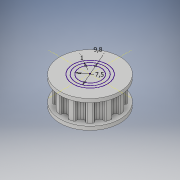
# Autodesk Inventor part: BeltPulleyT5_12Z
Saved by Autodesk Inventor 2018.3 (Build 223284000, 284)
## iProperties
Created: 2018-07-24
Part Number: BeltPulleyT5_12Z
Material: Generisch
Document SubType Name: Modeling
Designer: JochenAlt
Density: 1 g/cm^3
Appearance: Vorgabe
Author: JochenAlt
Autodesk Inventor part; units mm, degrees
ref_plane "YZ Plane" through (0, 0, 0) normal (1, 0, 0) x (0, 1, 0)
ref_plane "XZ Plane" through (0, 0, 0) normal (0, 1, 0) x (-1, 0, 0)
ref_plane "XY Plane" through (0, 0, 0) normal (0, 0, 1) x (1, 0, 0)
sketch "Skizze1" plane through (0, 0, 0) normal (0, 0, 1) x (1, 0, 0)
  circle A0 centre (0, 0) radius 3.75
  dimension "d0" = 7.5
  constraints: 1 centre point, 1 coincident
  measures "d0" diameter of A0
sketch "Skizze9" plane through (0, 0, 0) normal (1, 0, 0) x (0, 1, 0)
  line L0 (0, 0) -> (0, -14)
  line L1 (0, 0) -> (-10.325, 0)
  line L2 (-10.325, 0) -> (-10.325, -1.25)
  line L3 (-10.325, -1.25) -> (-9.125, -1.25)
  line L4 (-9.125, -1.25) -> (-9.125, -8.25)
  line L5 (-9.125, -8.25) -> (-10.325, -8.25)
  line L6 (-10.325, -8.25) -> (-10.325, -9.5)
  line L7 (-10.325, -9.5) -> (0, -9.5)
  line L8 (0, -9.5) -> (0, 0)
  dimension "d56" = 1.25
  dimension "d57" = 10.325
  dimension "d58" = 1.2
  dimension "d62" = 0
  dimension "d75" = 7
  constraints: 18 end point, 4 perpendicular, 2 collinear, 2 point on line, 2 vertical, 1 coincident, 1 horizontal, 1 parallel
  measures "d56" distance of L1.end L2.end
  measures "d57" distance of L0.start L1.end
  measures "d58" distance of L2.end L3.end
  measures "d62" distance between parallel lines of L0 L8
  measures "d75" distance of L3.end L4.end
revolve "Umdrehung5" add sketch "Skizze9" angle 360 about axis through (0, 0, 0) along (0, 0, -1)
sketch "Skizze10" plane through (0, 0, -1.25) normal (0, 0, -1) x (-1, 0, 0)
  circle A0 centre (0, 0) radius 36.5
  arc A1 (-8.9649, 1.7016) -> (-8.7088, 1.2512) centre (-8.572, 1.627) ccw
  line L0 (-8.7088, 1.2512) -> (-8.1066, 1.032)
  arc A2 (-7.7128, 0.4344) -> (-8.1066, 1.032) centre (-8.3118, 0.4682) ccw
  arc A3 (-7.7128, 0.4344) -> (-7.7128, -0.4344) centre (0, 0) ccw
  arc A4 (-8.1066, -1.032) -> (-7.7128, -0.4344) centre (-8.3118, -0.4682) ccw
  line L1 (-8.1066, -1.032) -> (-8.7088, -1.2512)
  arc A5 (-8.7088, -1.2512) -> (-8.9649, -1.7016) centre (-8.572, -1.627) ccw
  arc A6 (-8.9649, -1.7016) -> (-8.8141, -2.3617) centre (0, 0) ccw
  arc A7 (-8.8141, -2.3617) -> (-8.6147, -3.0088) centre (0, 0) ccw
  arc A8 (-8.6147, -3.0088) -> (-8.1676, -3.2708) centre (-8.237, -2.8769) ccw
  line L2 (-8.1676, -3.2708) -> (-7.5365, -3.1596)
  arc A9 (-6.8967, -3.4802) -> (-7.5365, -3.1596) centre (-7.4323, -3.7505) ccw
  arc A10 (-6.8967, -3.4802) -> (-6.4622, -4.2326) centre (0, 0) ccw
  arc A11 (-6.5045, -4.947) -> (-6.4622, -4.2326) centre (-6.9642, -4.5614) ccw
  line L3 (-6.5045, -4.947) -> (-6.9164, -5.4379)
  arc A12 (-6.9164, -5.4379) -> (-6.9131, -5.9561) centre (-6.61, -5.695) ccw
  arc A13 (-6.9131, -5.9561) -> (-6.4523, -6.4523) centre (0, 0) ccw
  arc A14 (-6.4523, -6.4523) -> (-5.9561, -6.9131) centre (0, 0) ccw
  arc A15 (-5.9561, -6.9131) -> (-5.4379, -6.9164) centre (-5.695, -6.61) ccw
  line L4 (-5.4379, -6.9164) -> (-4.947, -6.5045)
  arc A16 (-4.2326, -6.4622) -> (-4.947, -6.5045) centre (-4.5614, -6.9642) ccw
  arc A17 (-4.2326, -6.4622) -> (-3.4802, -6.8967) centre (0, 0) ccw
  arc A18 (-3.1596, -7.5365) -> (-3.4802, -6.8967) centre (-3.7505, -7.4323) ccw
  line L5 (-3.1596, -7.5365) -> (-3.2708, -8.1676)
  arc A19 (-3.2708, -8.1676) -> (-3.0088, -8.6147) centre (-2.8769, -8.237) ccw
  arc A20 (-3.0088, -8.6147) -> (-2.3617, -8.8141) centre (0, 0) ccw
  arc A21 (-2.3617, -8.8141) -> (-1.7016, -8.9649) centre (0, 0) ccw
  arc A22 (-1.7016, -8.9649) -> (-1.2512, -8.7088) centre (-1.627, -8.572) ccw
  line L6 (-1.2512, -8.7088) -> (-1.032, -8.1066)
  arc A23 (-0.4344, -7.7128) -> (-1.032, -8.1066) centre (-0.4682, -8.3118) ccw
  arc A24 (-0.4344, -7.7128) -> (0.4344, -7.7128) centre (0, 0) ccw
  arc A25 (1.032, -8.1066) -> (0.4344, -7.7128) centre (0.4682, -8.3118) ccw
  line L7 (1.032, -8.1066) -> (1.2512, -8.7088)
  arc A26 (1.2512, -8.7088) -> (1.7016, -8.9649) centre (1.627, -8.572) ccw
  arc A27 (1.7016, -8.9649) -> (2.3617, -8.8141) centre (0, 0) ccw
  arc A28 (2.3617, -8.8141) -> (3.0088, -8.6147) centre (0, 0) ccw
  arc A29 (3.0088, -8.6147) -> (3.2708, -8.1676) centre (2.8769, -8.237) ccw
  line L8 (3.2708, -8.1676) -> (3.1596, -7.5365)
  arc A30 (3.4802, -6.8967) -> (3.1596, -7.5365) centre (3.7505, -7.4323) ccw
  arc A31 (3.4802, -6.8967) -> (4.2326, -6.4622) centre (0, 0) ccw
  arc A32 (4.947, -6.5045) -> (4.2326, -6.4622) centre (4.5614, -6.9642) ccw
  line L9 (4.947, -6.5045) -> (5.4379, -6.9164)
  arc A33 (5.4379, -6.9164) -> (5.9561, -6.9131) centre (5.695, -6.61) ccw
  arc A34 (5.9561, -6.9131) -> (6.4523, -6.4523) centre (0, 0) ccw
  arc A35 (6.4523, -6.4523) -> (6.9131, -5.9561) centre (0, 0) ccw
  arc A36 (6.9131, -5.9561) -> (6.9164, -5.4379) centre (6.61, -5.695) ccw
  line L10 (6.9164, -5.4379) -> (6.5045, -4.947)
  arc A37 (6.4622, -4.2326) -> (6.5045, -4.947) centre (6.9642, -4.5614) ccw
  arc A38 (6.4622, -4.2326) -> (6.8967, -3.4802) centre (0, 0) ccw
  arc A39 (7.5365, -3.1596) -> (6.8967, -3.4802) centre (7.4323, -3.7505) ccw
  line L11 (7.5365, -3.1596) -> (8.1676, -3.2708)
  arc A40 (8.1676, -3.2708) -> (8.6147, -3.0088) centre (8.237, -2.8769) ccw
  arc A41 (8.6147, -3.0088) -> (8.8141, -2.3617) centre (0, 0) ccw
  arc A42 (8.8141, -2.3617) -> (8.9649, -1.7016) centre (0, 0) ccw
  arc A43 (8.9649, -1.7016) -> (8.7088, -1.2512) centre (8.572, -1.627) ccw
  line L12 (8.7088, -1.2512) -> (8.1066, -1.032)
  arc A44 (7.7128, -0.4344) -> (8.1066, -1.032) centre (8.3118, -0.4682) ccw
  arc A45 (7.7128, -0.4344) -> (7.7128, 0.4344) centre (0, 0) ccw
  arc A46 (8.1066, 1.032) -> (7.7128, 0.4344) centre (8.3118, 0.4682) ccw
  line L13 (8.1066, 1.032) -> (8.7088, 1.2512)
  arc A47 (8.7088, 1.2512) -> (8.9649, 1.7016) centre (8.572, 1.627) ccw
  arc A48 (8.9649, 1.7016) -> (8.8141, 2.3617) centre (0, 0) ccw
  arc A49 (8.8141, 2.3617) -> (8.6147, 3.0088) centre (0, 0) ccw
  arc A50 (8.6147, 3.0088) -> (8.1676, 3.2708) centre (8.237, 2.8769) ccw
  line L14 (8.1676, 3.2708) -> (7.5365, 3.1596)
  arc A51 (6.8967, 3.4802) -> (7.5365, 3.1596) centre (7.4323, 3.7505) ccw
  arc A52 (6.8967, 3.4802) -> (6.4622, 4.2326) centre (0, 0) ccw
  arc A53 (6.5045, 4.947) -> (6.4622, 4.2326) centre (6.9642, 4.5614) ccw
  line L15 (6.5045, 4.947) -> (6.9164, 5.4379)
  arc A54 (6.9164, 5.4379) -> (6.9131, 5.9561) centre (6.61, 5.695) ccw
  arc A55 (6.9131, 5.9561) -> (6.4523, 6.4523) centre (0, 0) ccw
  arc A56 (6.4523, 6.4523) -> (5.9561, 6.9131) centre (0, 0) ccw
  arc A57 (5.9561, 6.9131) -> (5.4379, 6.9164) centre (5.695, 6.61) ccw
  line L16 (5.4379, 6.9164) -> (4.947, 6.5045)
  arc A58 (4.2326, 6.4622) -> (4.947, 6.5045) centre (4.5614, 6.9642) ccw
  arc A59 (4.2326, 6.4622) -> (3.4802, 6.8967) centre (0, 0) ccw
  arc A60 (3.1596, 7.5365) -> (3.4802, 6.8967) centre (3.7505, 7.4323) ccw
  line L17 (3.1596, 7.5365) -> (3.2708, 8.1676)
  arc A61 (3.2708, 8.1676) -> (3.0088, 8.6147) centre (2.8769, 8.237) ccw
  arc A62 (3.0088, 8.6147) -> (2.3617, 8.8141) centre (0, 0) ccw
  arc A63 (2.3617, 8.8141) -> (1.7016, 8.9649) centre (0, 0) ccw
  arc A64 (1.7016, 8.9649) -> (1.2512, 8.7088) centre (1.627, 8.572) ccw
  line L18 (1.2512, 8.7088) -> (1.032, 8.1066)
  arc A65 (0.4344, 7.7128) -> (1.032, 8.1066) centre (0.4682, 8.3118) ccw
  arc A66 (0.4344, 7.7128) -> (-0.4344, 7.7128) centre (0, 0) ccw
  arc A67 (-1.032, 8.1066) -> (-0.4344, 7.7128) centre (-0.4682, 8.3118) ccw
  line L19 (-1.032, 8.1066) -> (-1.2512, 8.7088)
  arc A68 (-1.2512, 8.7088) -> (-1.7016, 8.9649) centre (-1.627, 8.572) ccw
  arc A69 (-1.7016, 8.9649) -> (-2.3617, 8.8141) centre (0, 0) ccw
  arc A70 (-2.3617, 8.8141) -> (-3.0088, 8.6147) centre (0, 0) ccw
  arc A71 (-3.0088, 8.6147) -> (-3.2708, 8.1676) centre (-2.8769, 8.237) ccw
  line L20 (-3.2708, 8.1676) -> (-3.1596, 7.5365)
  arc A72 (-3.4802, 6.8967) -> (-3.1596, 7.5365) centre (-3.7505, 7.4323) ccw
  arc A73 (-3.4802, 6.8967) -> (-4.2326, 6.4622) centre (0, 0) ccw
  arc A74 (-4.947, 6.5045) -> (-4.2326, 6.4622) centre (-4.5614, 6.9642) ccw
  line L21 (-4.947, 6.5045) -> (-5.4379, 6.9164)
  arc A75 (-5.4379, 6.9164) -> (-5.9561, 6.9131) centre (-5.695, 6.61) ccw
  arc A76 (-5.9561, 6.9131) -> (-6.4523, 6.4523) centre (0, 0) ccw
  arc A77 (-6.4523, 6.4523) -> (-6.9131, 5.9561) centre (0, 0) ccw
  arc A78 (-6.9131, 5.9561) -> (-6.9164, 5.4379) centre (-6.61, 5.695) ccw
  line L22 (-6.9164, 5.4379) -> (-6.5045, 4.947)
  arc A79 (-6.4622, 4.2326) -> (-6.5045, 4.947) centre (-6.9642, 4.5614) ccw
  arc A80 (-6.4622, 4.2326) -> (-6.8967, 3.4802) centre (0, 0) ccw
  arc A81 (-7.5365, 3.1596) -> (-6.8967, 3.4802) centre (-7.4323, 3.7505) ccw
  line L23 (-7.5365, 3.1596) -> (-8.1676, 3.2708)
  arc A82 (-8.1676, 3.2708) -> (-8.6147, 3.0088) centre (-8.237, 2.8769) ccw
  arc A83 (-8.6147, 3.0088) -> (-8.8141, 2.3617) centre (0, 0) ccw
  arc A84 (-8.8141, 2.3617) -> (-8.9649, 1.7016) centre (0, 0) ccw
  constraints: 168 point on circle, 85 centre point, 48 end point
extrude "Extrusion3" cut sketch "Skizze10" along normal up to surface (7 mm away)
sketch "Skizze11" plane through (0, 0, 0) normal (0, 0, 1) x (1, 0, 0)
  line L0 (0, 14.455) -> (0, -14.455) construction
  line L1 (-14.455, 0) -> (14.455, 0) construction
  circle A0 centre (0, 0) radius 4.9
  circle A1 centre (0, 0) radius 5.9
  dimension "d63" = 9.8
  dimension "d66" = 1
  constraints: 2 centre point, 2 coincident
  measures "d63" diameter of A0
  measures "d66" radial gap between concentric circles of A1 A0
equation "\"d19\" = 60deg"
equation "\"Skizze2_Pitch\" = 3"
equation "\"d38\" = 60deg"
equation "\"Skizze6_Pitch\" = 2"
equation "\"d83\" = 60deg"
equation "\"Skizze12_Pitch\" = 2"
equation "\"d102\" = 60deg"
equation "\"Skizze15_Pitch\" = 1.81429"
equation "\"d121\" = 60deg"
equation "\"Skizze19_Pitch\" = 2.30909"
equation "\"d140\" = 60deg"
equation "\"Skizze23_Pitch\" = 2.30909"
equation "\"d163\" = 60deg"
equation "\"Skizze26_Pitch\" = 2.30909"
